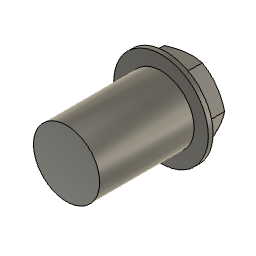
A1_AI22BTECH11005_2 (Autodesk Fusion 360 design; units mm, degrees)
Autodesk Fusion 360 part; units mm, degrees
sketch "Sketch1" plane through (0, 0, 0) normal (0, 1, 0) x (1, 0, 0)
  line L0 (4.0197, -0.419) -> (2.3727, 3.2717)
  line L1 (2.3727, 3.2717) -> (-1.647, 3.6906)
  line L2 (-1.647, 3.6906) -> (-4.0197, 0.419)
  line L3 (-4.0197, 0.419) -> (-2.3727, -3.2717)
  line L4 (-2.3727, -3.2717) -> (1.647, -3.6906)
  line L5 (1.647, -3.6906) -> (4.0197, -0.419)
  circle A0 centre (0, 0) radius 3.5
  dimension "d2" = 7
  constraint coincident A0.centre origin
  measures "d2" diameter of A0
extrude "Extrude1" add sketch "Sketch1" along normal blind 2.5
sketch "Sketch2" plane through (0, 0, 0) normal (0, 1, 0) x (1, 0, 0)
  circle A0 centre (0, 0) radius 5
  dimension "d5" = 10
  constraint coincident A0.centre origin
  measures "d5" diameter of A0
extrude "Extrude2" add sketch "Sketch2" against normal blind 0.5
sketch "Sketch3" plane through (0, 2.5, 0) normal (0, 1, 0) x (-1, 0, 0)
  line L0 (-1.647, 3.6906) -> (-4.0197, 0.419)
  line L1 (-4.0197, 0.419) -> (-2.3727, -3.2717)
  line L2 (-2.3727, -3.2717) -> (1.647, -3.6906)
  line L3 (1.647, -3.6906) -> (4.0197, -0.419)
  line L4 (4.0197, -0.419) -> (2.3727, 3.2717)
  line L5 (2.3727, 3.2717) -> (-1.647, 3.6906)
  circle A0 centre (0, 0) radius 3.5
  dimension "d8" = 7
  constraint coincident A0.centre origin
  measures "d8" diameter of A0
extrude "Extrude3" add sketch "Sketch3" against normal blind 13 contours A0
sketch "Sketch4" plane through (0, 2.5, 0) normal (0, 1, 0) x (-1, 0, 0)
ref_plane "WorkPlane1" through (0, 1.25, 0) normal (-0.10367, 0, 0.994612) x (0.994612, 0, 0.10367)
sketch "Sketch5" plane through (0, 1.25, 0) normal (-0.10367, 0, 0.994612) x (0.994612, 0, 0.10367)
  line L0 (0, 0) -> (0, 1.25)
  constraint coincident L0.start origin
  constraint vertical L0
sketch "Sketch6" plane through (0, 1.25, 0) normal (-0.10367, 0, 0.994612) x (0.994612, 0, 0.10367)
sketch "Sketch7" plane through (0, 1.25, 0) normal (-0.10367, 0, 0.994612) x (0.994612, 0, 0.10367)
  line L0 (4.0463, 1.2672) -> (3.5, 1.2672)
  line L1 (4.0463, 1.2672) -> (4.0463, 0.9519)
  line L2 (3.5, 1.2672) -> (4.0463, 0.9519)
  line L3 (0, 6.5) -> (0, -6)
  constraint horizontal L0
  constraint perpendicular L0 L1
revolve "Revolve1" cut sketch "Sketch7" angle 360 about axis through (0, 7.75, 0) along (0, -1, 0)
